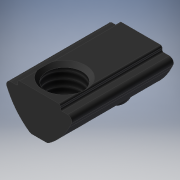
# Autodesk Inventor part: 13084_m
Saved by Autodesk Inventor 2025 (Build 290162000, 162)
## iProperties
Created: 2024-07-17
Part Number: 13084_m
Material: Generic
Catalog Web Link: www.cadenas.de
Description: 13082, 13083, 13084, 13027, 13028, 13031, 13034, 13039, 13037, 13040, 13029, 13032, 13035_m-Roll-In T-Nuts with Ball Spring
Vendor: 8020
Document SubType Name: Modeling
Designer: psAdmin
Manufacturer: 8020
Mass: 0.24598 g
Surface Area: 3.77442 cm^2
Volume: 0.24598 cm^3
Density: 1 g/cm^3
Appearance: PSOLRGB-175-175-175
Category: PARTsolutions
Company: 8020
PSOL_IDENT_0: {$CADENAS_DATA/23d-libs/8020/metric/fastening_options/13082_m.prj},242 {VTYP=3D},{NB=13084_m},{LINA=
PSOL_IDENT_1: 13084},{NN=13082, 13083, 13084, 13027, 13028, 13031, 13034, 13039, 13037, 13040, 13029, 13032, 13035
PSOL_IDENT_2: _m},{DATE=27.07.2023 19:29:46},{GEOMDATE=27.06.2019 19:54:57},{VERSION=},{LINEID=10},{WBVAR=MAT,A},{
PSOL_IDENT_3: WBNUMERIC=}  {NB=13084_m},{LINA=13084},{KT=DUMMY},{PN=13084},{MAT=1},{MAT1= '1','Steel' },{FIN=Zinc
PSOL_IDENT_4: Plated},{A=M5},{A1= 'M3','M3','M4','M4','M5','M5' },{A2=5.0000},{B=12.00},{C=7.69},{D=4.70},{E=5.00}
PSOL_IDENT_5: ,{F=0.60},{G=0.85},{W=.0018},{CC=5-20},{TT=M},{NO=1},{C1=7.700},{R1=0.20},{R2=0.50},{R3=7.50},{R4=1.
PSOL_IDENT_6: 50},{B1=3.00},{E1=2.00}
NB: 13084_m
NN: 13082, 13083, 13084, 13027, 13028, 13031, 13034, 13039, 13037, 13040, 13029, 13032, 13035_m
NT: Roll-In T-Nuts with Ball Spring
NBSYN: $PN._m
LINA: 13084
CATALOG: 80/20
PN: 13084
MAT: Steel
FIN: Zinc Plated
A: M5
B: 12
C: 7.69
D: 4.7
E: 5
F: 0.6
G: 0.85
W: .0018
CC: 5-20
SUPPLIER: 8020
ARTICLENO: 13084_m
BOMINFO: 13084
CREATOR: CADENAS GmbH
Title: 13084
Author: Cadenas PARTsolutions
Comments: Roll-In T-Nuts with Ball Spring
Autodesk Inventor part; units mm, degrees
sketch "Sketch_1" plane through (0, 0, 0) normal (0, 0, 1) x (1, 0, 0)
  arc A0 (-3.35, 0) -> (-3.7968, -0.7244) centre (-3.35, -0.5) ccw
  line L0 (-3.7968, -0.7244) -> (-3.5468, -1.2222)
  arc A1 (-3.5468, -1.2222) -> (-1.1318, -4.0103) centre (3.1555, 2.1435) ccw
  arc A2 (-1.1318, -4.0103) -> (-0.846, -4.1) centre (-0.846, -3.6) ccw
  line L1 (-0.846, -4.1) -> (0.846, -4.1)
  arc A3 (0.846, -4.1) -> (1.1318, -4.0103) centre (0.846, -3.6) ccw
  arc A4 (1.1318, -4.0103) -> (3.5468, -1.2222) centre (-3.1555, 2.1435) ccw
  line L2 (3.5468, -1.2222) -> (3.7968, -0.7244)
  arc A5 (3.7968, -0.7244) -> (3.35, 0) centre (3.35, -0.5) ccw
  line L3 (3.35, 0) -> (2.7, 0)
  arc A6 (2.5, 0.2) -> (2.7, 0) centre (2.7, 0.2) ccw
  line L4 (2.5, 0.2) -> (2.5, 0.4)
  arc A7 (2.5, 0.4) -> (2.3, 0.6) centre (2.3, 0.4) ccw
  line L5 (2.3, 0.6) -> (-2.3, 0.6)
  arc A8 (-2.3, 0.6) -> (-2.5, 0.4) centre (-2.3, 0.4) ccw
  line L6 (-2.5, 0.4) -> (-2.5, 0.2)
  arc A9 (-2.7, 0) -> (-2.5, 0.2) centre (-2.7, 0.2) ccw
  line L7 (-2.7, 0) -> (-3.35, 0)
  constraints: 20 point on circle, 16 end point, 10 centre point
extrude "Extrusion1" add sketch "Sketch_1" along normal mid plane 12
sketch "Sketch_2" plane through (0, 0, 0) normal (1, 0, 0) x (0, 1, 0)
  line L0 (0.6, 3) -> (-4.1, 3)
  line L1 (-4.1, 3) -> (-4.1, 5.5)
  line L2 (-4.1, 5.5) -> (-3.667, 5.067)
  line L3 (-3.667, 5.067) -> (0.167, 5.067)
  line L4 (0.167, 5.067) -> (0.6, 5.5)
  line L5 (0.6, 5.5) -> (0.6, 3)
  line L6 (0.6, 3) -> (-4.1, 3)
  constraints: 14 end point
revolve "Revolution1" cut sketch "Sketch_2" angle 360 about axis through (0, 0.6, 3) along (0, 1, 0)
thread "Thread1" size "M5x0.8" class "6H" standard "ISO Metric profile" full length
sketch "Sketch3" plane through (-0.846, -4.1, -6) normal (0, -1, 0) x (1, 0, 0)
  point P0 (0.846, 3)
hole "Hole1" at (0, -4.1, -3) direction (0, 1, 0) diameter 3 depth 3.28
sketch "Sketch_5" plane through (0, 0, 0) normal (1, 0, 0) x (0, 1, 0)
  line L0 (-3.449, -1.499) -> (-3.449, -4.501)
  arc A0 (-3.449, -1.499) -> (-3.449, -4.501) centre (-3.449, -3) ccw
  line L1 (-3.449, -1.499) -> (-3.449, -4.501)
  constraints: 4 end point, 2 point on circle, 1 centre point
revolve "Revolution2" add sketch "Sketch_5" angle 360 about axis through (0, -3.449, -1.499) along (0, 0, 1)
ref_plane "nut_to_bolt_XY" through (0, 0, 3) normal (0, 1, 0) x (1, 0, 0)
ref_plane "nut_to_bolt_YZ" through (0, 0, 3) normal (1, 0, 0) x (0, 0, -1)
ref_plane "nut_to_bolt_ZX" through (0, 0, 3) normal (0, 0, -1) x (0, 1, 0)
body "Solid1"
